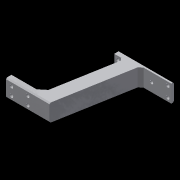
# Autodesk Inventor part: AXLG
Saved by Autodesk Inventor 2016 (Build 200138000, 138)
## iProperties
Created: 2017-08-21
Part Number: AXLG
Material: PC/ABS Plastic
Document SubType Name: Modeling
Designer: ludwi
Density: 0.357273 g/cm^3
Appearance: Smooth - White
Author: ludwi
Autodesk Inventor part; units mm, degrees
ref_plane "YZ Plane" through (0, 0, 0) normal (1, 0, 0) x (0, 1, 0)
ref_plane "XZ Plane" through (0, 0, 0) normal (0, 1, 0) x (-1, 0, 0)
ref_plane "XY Plane" through (0, 0, 0) normal (0, 0, 1) x (1, 0, 0)
sketch "Sketch1" plane through (0, 0, 0) normal (0, 0, 1) x (1, 0, 0)
  line L0 (483.5261, -135.8063) -> (507.8593, 2.1937)
  line L1 (509.6225, 12.1937) -> (464.6225, 12.1937)
  line L2 (464.6225, 14.1937) -> (464.6225, 12.1937) construction
  line L3 (464.6225, 12.1937) -> (564.6225, 12.1937) construction
  line L4 (564.6225, 12.1937) -> (564.6225, 14.1937) construction
  line L5 (564.6225, 14.1937) -> (464.6225, 14.1937) construction
  line L6 (564.6225, 14.1937) -> (464.6225, 14.1937) construction
  line L7 (564.6225, 14.1937) -> (564.6225, 30.1937) construction
  line L8 (552.6225, 30.1937) -> (564.6225, 30.1937) construction
  arc A0 (536.6225, 30.1937) -> (552.6225, 30.1937) centre (544.6225, 30.1937) ccw construction
  line L9 (527.1225, 30.1937) -> (536.6225, 30.1937) construction
  arc A1 (502.1225, 30.1937) -> (527.1225, 30.1937) centre (514.6225, 30.1937) ccw construction
  line L10 (492.6225, 30.1937) -> (502.1225, 30.1937) construction
  arc A2 (476.6225, 30.1937) -> (492.6225, 30.1937) centre (484.6225, 30.1937) ccw construction
  line L11 (464.6225, 30.1937) -> (476.6225, 30.1937) construction
  line L12 (464.6225, 14.1937) -> (464.6225, 30.1937) construction
  line L13 (464.6225, 12.1937) -> (464.6225, 2.1937)
  line L14 (464.6225, 2.1937) -> (482.4736, 2.1937)
  line L15 (482.4736, 2.1937) -> (459.9038, -125.8063)
  line L16 (564.6225, 12.1937) -> (464.6225, 12.1937)
  line L17 (464.6225, 12.1937) -> (464.6225, 7.1937)
  line L18 (483.5261, -135.8063) -> (403.5261, -135.8063)
  line L19 (403.5261, -135.8063) -> (403.5261, -125.8063)
  line L20 (403.5261, -125.8063) -> (459.9038, -125.8063)
  line L21 (507.8593, 2.1937) -> (564.6225, 2.1937)
  line L22 (564.6225, 2.1937) -> (564.6225, 12.1937)
  point P0 (0, 0)
  dimension "d16" = 45
  dimension "d17" = 25
  dimension "d25" = 10
  dimension "d26" = 80
  dimension "d58" = 80
  dimension "d59" = 10
  dimension "d62" = 150
  constraints: 24 end point, 5 horizontal, 4 perpendicular, 1 midpoint, 1 parallel, 1 vertical
  measures "d16" distance of L1.end L1.start
  measures "d17" distance between parallel lines of L0 L15
  measures "d25" distance of L1.end L13.end
  measures "d26" angle of L1 L0
  measures "d58" distance of L0.start L18.end
  measures "d59" distance of L18.end L19.end
  measures "d62" distance between parallel lines of L18 L5
extrude "Extrusion1" add sketch "Sketch1" against normal blind 32
chamfer "Chamfer5" distance 5 angle 45 1 edges at (507.8593, 2.1937, -16)
chamfer "Chamfer8" distance 5 angle 45 1 edges at (482.4736, 2.1937, -16)
chamfer "Chamfer11" distance 8 angle 45 1 edges at (459.9038, -125.8063, -16)
chamfer "Chamfer6" distance 2 angle 45 10 edges at (443.5261, -135.8063, 0) (443.5261, -135.8063, -32) (514.6225, 12.1937, 0) (514.6225, 12.1937, -32) (538.7409, 2.1937, -32) (538.7409, 2.1937, 0) (471.0481, 2.1937, -32) (471.0481, 2.1937, 0) (427.715, -125.8063, -32) (427.715, -125.8063, 0)
sketch "Sketch9" plane through (464.6225, 12.1937, -2) normal (0, 1, 0) x (1, 0, 0)
  circle A0 centre (6.5, 23.5) radius 3.2
  circle A1 centre (6.5, 4.5) radius 3.2
  circle A2 centre (36.3, 14) radius 3
  circle A3 centre (63.7, 14) radius 3
  circle A4 centre (93.5, 23.5) radius 3.2
  circle A5 centre (93.5, 4.5) radius 3.2
  point P0 (-464.6225, -2)
  constraints: 6 centre point, 12 other
extrude "Extrusion6" cut sketch "Sketch9" against normal blind 32 contours A0 | A1 | A3 | A4 | A5
sketch "Sketch10" plane through (403.5261, -135.8063, -30) normal (0, -1, 0) x (1, 0, 0)
  line L0 (80, 28) -> (80, 0) projected
  line L1 (0, 28) -> (0, 0) projected
  circle A0 centre (10, 21.5) radius 3.2
  circle A1 centre (10, 6.5) radius 3.2
  circle A2 centre (40, 21.5) radius 3.2
  circle A3 centre (40, 6.5) radius 3.2
  line L2 (10, 21.5) -> (40, 21.5) construction
  line L3 (40, 21.5) -> (40, 6.5) construction
  line L4 (40, 6.5) -> (10, 6.5) construction
  line L5 (10, 6.5) -> (10, 21.5) construction
  line L6 (80, 0) -> (0, 0) projected
  line L7 (0, 28) -> (80, 28) projected
  point P0 (-403.5261, 30)
  point P1 (10, 14)
  point P2 (0, 14)
  dimension "d51" = 6.4
  dimension "d52" = 10
  dimension "d53" = 30
  dimension "d54" = 15
  constraints: 8 end point, 4 centre point, 3 equal radius, 2 coincident, 2 midpoint, 2 parallel, 1 horizontal, 1 horizontal alignment, 1 perpendicular
  measures "d51" diameter of A2
  measures "d52" distance between parallel lines of L1 L5
  measures "d53" distance of L2.start L2.end
  measures "d54" distance of L4.end L2.start
extrude "Extrusion7" cut sketch "Sketch10" against normal blind 32 contours A0 | A1 | A2 | A3
chamfer "Chamfer10" distance 2.5 angle 45 4 edges at (440.3261, -125.8063, -23.5) (440.3261, -125.8063, -8.5) (410.3261, -125.8063, -23.5) (410.3261, -125.8063, -8.5)
body "Solid1"
